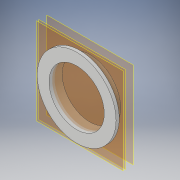
# Autodesk Inventor part: KF50tube_v2
Saved by Autodesk Inventor 2018 (Build 220112000, 112)
## iProperties
Created: 2017-06-29
Part Number: KF50tube_v2
Material: Generic
Document SubType Name: Modeling
Designer: boss
Density: 1 g/cm^3
Appearance: Default
Author: boss
Autodesk Inventor part; units mm, degrees
ref_plane "YZ Plane" through (0, 0, 0) normal (1, 0, 0) x (0, 1, 0)
ref_plane "XZ Plane" through (0, 0, 0) normal (0, 1, 0) x (-1, 0, 0)
sketch "Sketch1" plane through (0, 0, 0) normal (0, 0, 1) x (1, 0, 0)
  circle A0 centre (0, 0) radius 37.465
  dimension "d0" = 74.93
  constraints: 1 centre point, 1 coincident
  measures "d0" diameter of A0
extrude "Extrusion1" add sketch "Sketch1" along normal blind 25.4
sketch "Sketch3" plane through (0, 0, 25.4) normal (0, 0, 1) x (1, 0, 0)
  circle A0 centre (0, 0) radius 26.289
  dimension "d6" = 52.578
  constraints: 1 centre point, 1 coincident
  measures "d6" diameter of A0
extrude "Extrusion3" cut sketch "Sketch3" against normal blind 2.54
sketch "Sketch4" plane through (0, 0, 0) normal (0, 0, -1) x (-1, 0, 0)
  circle A0 centre (0, 0) radius 26.289
  dimension "d9" = 52.578
  constraints: 1 centre point, 1 coincident
  measures "d9" diameter of A0
extrude "Extrusion4" cut sketch "Sketch4" against normal blind 2.54
ref_plane "Work Plane1" through (0, 0, 12.7) normal (0, 0, 1) x (1, 0, 0)
sketch "Sketch5" plane through (0, 0, 12.7) normal (0, 0, 1) x (1, 0, 0)
  circle A0 centre (0, 0) radius 29.337
  circle A1 centre (0, 0) radius 37.465
  dimension "d13" = 58.674
  dimension "d34" = 74.93
  constraints: 2 centre point, 2 coincident
  measures "d13" diameter of A0
  measures "d34" diameter of A1
extrude "Extrusion5" cut sketch "Sketch5" along normal mid plane 19.304
ref_plane "Work Plane2" through (0, 0, 20.1676) normal (0, 0, 1) x (1, 0, 0)
sketch "Sketch6" plane through (0, 0, 20.1676) normal (0, 0, 1) x (1, 0, 0)
  circle A0 centre (0, 0) radius 29.337
  dimension "d17" = 58.674
  constraints: 1 centre point, 1 coincident
  measures "d17" diameter of A0
loft "Loft1" add profiles "Sketch6" section 1 edges at (-37.465, 0, 22.352)
ref_plane "Work Plane3" through (0, 0, 5.2324) normal (0, 0, 1) x (1, 0, 0)
sketch "Sketch7" plane through (0, 0, 5.2324) normal (0, 0, 1) x (1, 0, 0)
  circle A0 centre (0, 0) radius 29.337
  dimension "d31" = 58.674
  constraints: 1 centre point, 1 coincident
  measures "d31" diameter of A0
loft "Loft3" add profiles "Sketch7" section 1 edges at (-37.465, 0, 3.048)
sketch "Sketch2" plane through (0, 0, 25.4) normal (0, 0, 1) x (1, 0, 0)
  circle A0 centre (0, 0) radius 26.289
  dimension "d3" = 52.578
  constraints: 1 centre point, 1 coincident
  measures "d3" diameter of A0
extrude "Extrusion2" cut sketch "Sketch2" against normal blind 50.8
ref_plane "Work Plane4" through (0, 0, 22.352) normal (0, 0, 1) x (1, 0, 0)
ref_plane "Work Plane5" through (0, 0, 3.048) normal (0, 0, 1) x (1, 0, 0)
body "Solid1"
